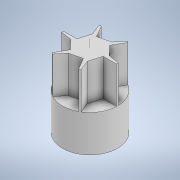
# Autodesk Inventor part: test
Saved by Autodesk Inventor 2021 (Build 250183000, 183)
## iProperties
Created: 2020-06-19
Part Number: test
Material: Generic
Document SubType Name: Modeling
Designer: robst
Density: 1 g/cm^3
Appearance: Default
Author: robst
Autodesk Inventor part; units mm, degrees
ref_plane "YZ Plane" through (0, 0, 0) normal (1, 0, 0) x (0, 1, 0)
ref_plane "XZ Plane" through (0, 0, 0) normal (0, 1, 0) x (-1, 0, 0)
ref_plane "XY Plane" through (0, 0, 0) normal (0, 0, 1) x (1, 0, 0)
sketch "Sketch1" plane through (0, 0, 0) normal (0, 1, 0) x (-1, 0, 0)
  circle A0 centre (0, 0) radius 9.525
  dimension "d0" = 19.05
  constraints: 1 centre point, 1 coincident
  measures "d0" diameter of A0
extrude "Extrusion1" add sketch "Sketch1" along normal blind 25.4
sketch "Sketch2" plane through (0, 25.4, 0) normal (0, 1, 0) x (1, 0, 0)
  arc A0 (4.4938, 8.3983) -> (-4.4938, 8.3983) centre (0, 0) ccw
  line L0 (-4.4938, 8.3983) -> (-2.1272, 4.4011)
  line L1 (-2.1272, 4.4011) -> (2.1272, 5.428)
  line L2 (2.1272, 5.428) -> (4.4938, 8.3983)
  constraints: 6 end point, 2 point on circle, 1 centre point, 1 coincident
extrude "Extrusion2" cut sketch "Sketch2" against normal blind 12.7
pattern_circular "Circular Pattern1" count 6 over 360 about axis through (0, -10, 0) along (0, 1, 0) of "Extrusion2"
body "Solid1"
